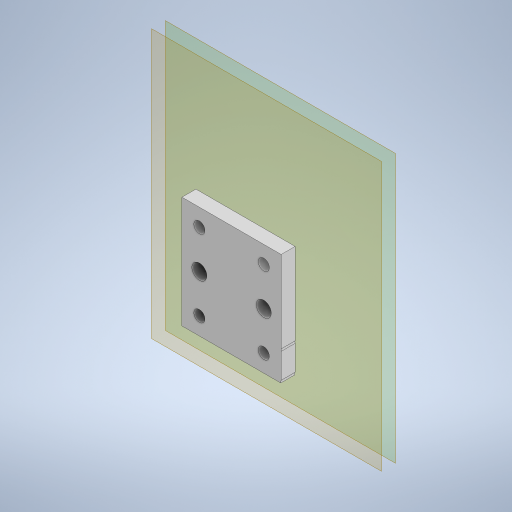
# Autodesk Inventor part: полное крепление каретки
Saved by Autodesk Inventor 2024.2 (Build 282272000, 272)
## iProperties
Created: 2026-01-10
Part Number: полное крепление каретки
Material: Типовые
Document SubType Name: Modeling
Designer: Service
Density: 1 g/cm^3
Appearance: По умолчанию
Author: Service
Autodesk Inventor part; units mm, degrees
ref_plane "YZ Plane" through (0, 0, 0) normal (1, 0, 0) x (0, 1, 0)
ref_plane "XZ Plane" through (0, 0, 0) normal (0, 1, 0) x (-1, 0, 0)
ref_plane "XY Plane" through (0, 0, 0) normal (0, 0, 1) x (1, 0, 0)
ref_plane "РабПлоскость1" through (0, 0, -4) normal (0, 0, -1) x (-1, 0, 0)
ref_plane "РабПлоскость2" through (0, 0, 0) normal (0, 0, 1) x (1, 0, 0)
sketch "Эскиз2" plane through (0, 0, 0) normal (0, 0, 1) x (1, 0, 0)
  line L0 (-17.8008, -6.6339) -> (10.6717, -6.6339)
  line L1 (10.6717, -6.6339) -> (10.6717, 25.3661)
  line L2 (10.6717, 25.3661) -> (-17.8008, 25.3661)
  line L3 (-17.8008, 25.3661) -> (-17.8008, -6.6339)
  circle A0 centre (-31.4768, 2.1354) radius 0.9
  circle A1 centre (23.5157, 1.4536) radius 0.9
  circle A2 centre (-19.4778, 1.9866) radius 0.9
  circle A3 centre (-19.5769, -6.0128) radius 0.9
  circle A4 centre (23.4165, -6.5458) radius 0.9
  circle A5 centre (11.5166, 1.6023) radius 0.9
  circle A6 centre (11.4174, -6.3971) radius 0.9
  circle A7 centre (-31.576, -5.864) radius 0.9
  circle A8 centre (-12.8008, -1.6339) radius 1.6
  circle A9 centre (5.6717, -1.6339) radius 1.6
  circle A10 centre (-12.8008, 20.3661) radius 1.6
  circle A11 centre (5.6717, 20.3661) radius 1.6
  arc A12 (11.4355, 36.4061) -> (11.4355, 44.3661) centre (11.4355, 40.3861) ccw
  line L4 (11.4355, 44.3661) -> (-18.5645, 44.3661)
  arc A13 (-18.5645, 44.3661) -> (-18.5645, 36.4061) centre (-18.5645, 40.3861) ccw
  line L5 (-18.5645, 36.4061) -> (11.4355, 36.4061)
  line L6 (-33.5645, -20.6339) -> (-33.5645, 49.3661)
  line L7 (-33.5645, 49.3661) -> (26.4355, 49.3661)
  line L8 (26.4355, 49.3661) -> (26.4355, -20.6339)
  line L9 (26.4355, -20.6339) -> (-33.5645, -20.6339)
  circle A14 centre (-12.8008, 9.3661) radius 2.15
  circle A15 centre (5.6717, 9.3661) radius 2.15
  point P0 (0, 0)
  point P1 (-17.8008, 9.3661)
  point P2 (10.5491, -6.6339)
  point P3 (10.6717, -5.8931)
  point P4 (10.6717, 1.2922)
  point P5 (10.6717, 1.9125)
  dimension "d0" = 5
  dimension "d1" = 5
  dimension "d2" = 5
  dimension "d3" = 5
  dimension "d4" = 4.3
  dimension "d5" = 4.3
  dimension "d6" = 16
  dimension "d7" = 5
  dimension "d8" = 16
  dimension "d9" = 5
  constraints: 20 end point, 16 centre point, 5 horizontal, 4 point on circle, 2 parallel, 2 vertical, 1 midpoint, 1 perpendicular, 36 other
  measures "d0" distance from line of L3 A10.centre
  measures "d1" distance from line of L0 A8.centre
  measures "d2" distance from line of L1 A9.centre
  measures "d3" distance from line of L2 A11.centre
  measures "d4" diameter of A15
  measures "d5" diameter of A14
  measures "d6" distance from line of L2 A14.centre
  measures "d7" distance from line of L1 A15.centre
  measures "d8" distance from line of L0 A15.centre
  measures "d9" distance of point (-17.801, 9.366) A14.centre
extrude "Выдавливание1" add sketch "Эскиз2" along normal blind 10 contours L3 L2 L1 A5 A6 L0 | A14 | A15
sketch "Эскиз3" plane through (0, 0, 10) normal (0, 0, 1) x (1, 0, 0)
  circle A0 centre (-12.8008, 9.3661) radius 2.15
  circle A1 centre (5.6717, 9.3661) radius 2.15
  line L0 (10.6717, 1.9125) -> (10.6717, 25.3661) projected
  line L1 (10.6717, 25.3661) -> (-17.8008, 25.3661) projected
  line L2 (-17.8008, 25.3661) -> (-17.8008, -6.6339) projected
  point P0 (0, 0)
  dimension "d12" = 5
  dimension "d13" = 16
  dimension "d14" = 5
  dimension "d15" = 16
  dimension "d16" = 4.3
  dimension "d17" = 4.3
  constraints: 2 centre point
  measures "d12" distance from line of L0 A1.centre
  measures "d13" distance from line of L1 A1.centre
  measures "d14" distance from line of L2 A0.centre
  measures "d15" distance from line of L1 A0.centre
  measures "d16" diameter of A0
  measures "d17" diameter of A1
extrude "Выдавливание2" cut sketch "Эскиз3" against normal blind 4
sketch "Эскиз4" plane through (-12.8008, 9.3661, 6) normal (0, 0, 1) x (1, 0, 0)
  line L0 (-12.8791, 27.3861) -> (32.0773, 27.3861)
  line L1 (32.0773, 27.3861) -> (32.0773, -22.3728)
  line L2 (32.0773, -22.3728) -> (-12.8791, -22.3728)
  line L3 (-12.8791, -22.3728) -> (-12.8791, 27.3861)
  point P0 (12.8008, -9.3661)
  constraints: 8 end point, 2 parallel, 1 horizontal, 1 perpendicular
extrude "Выдавливание3" cut sketch "Эскиз4" against normal blind 10
